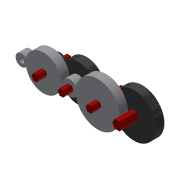
# Autodesk Inventor part: MultiStage Gearbox Sketch Double File
Saved by Autodesk Inventor 2013 (Build 170138000, 138)
## iProperties
Created: 2014-01-26
Part Number: MultiStage Gearbox Sketch Double File
Material: Generic
Document SubType Name: Modeling
Designer: Nemo
Density: 1 g/cm^3
Author: Nemo
Autodesk Inventor part; units mm, degrees
ref_plane "YZ Plane" through (0, 0, 0) normal (1, 0, 0) x (0, 1, 0)
ref_plane "XZ Plane" through (0, 0, 0) normal (0, 1, 0) x (-1, 0, 0)
ref_plane "XY Plane" through (0, 0, 0) normal (0, 0, 1) x (1, 0, 0)
sketch "Sketch1" plane through (0, 0, 0) normal (0, 0, 1) x (1, 0, 0)
  circle A0 centre (0, 0) radius 26.67
  line L0 (5.4993, 0) -> (2.7496, -4.7625)
  line L1 (2.7496, -4.7625) -> (-2.7496, -4.7625)
  line L2 (-2.7496, -4.7625) -> (-5.4993, 0)
  line L3 (-5.4993, 0) -> (-2.7496, 4.7625)
  line L4 (-2.7496, 4.7625) -> (2.7496, 4.7625)
  line L5 (2.7496, 4.7625) -> (5.4993, 0)
  circle A1 centre (0, 0) radius 13.97
  circle A2 centre (39.4462, 0) radius 27.94
  circle A3 centre (39.4462, 0) radius 11.43
  circle A4 centre (-33.0962, 0) radius 8.89
  circle A5 centre (81.4324, 0) radius 33.02
  line L6 (78.6828, 4.7625) -> (84.182, 4.7625)
  line L7 (84.182, 4.7625) -> (86.9317, 0)
  line L8 (86.9317, 0) -> (84.182, -4.7625)
  line L9 (84.182, -4.7625) -> (78.6828, -4.7625)
  line L10 (78.6828, -4.7625) -> (75.9331, 0)
  line L11 (75.9331, 0) -> (78.6828, 4.7625)
  line L12 (33.9469, 0) -> (36.6966, 4.7625)
  line L13 (36.6966, 4.7625) -> (42.1958, 4.7625)
  line L14 (42.1958, 4.7625) -> (44.9455, 0)
  line L15 (44.9455, 0) -> (42.1958, -4.7625)
  line L16 (42.1958, -4.7625) -> (36.6966, -4.7625)
  line L17 (36.6966, -4.7625) -> (33.9469, 0)
  circle A6 centre (-33.0962, 0) radius 4
  line L18 (-34.0962, 4.873) -> (-32.0962, 4.873)
  line L19 (-32.0962, 4.873) -> (-32.0962, 2.873)
  line L20 (-32.0962, 2.873) -> (-34.0962, 2.873)
  line L21 (-34.0962, 2.873) -> (-34.0962, 4.873)
  circle A7 centre (81.4324, 0) radius 11.43
  circle A8 centre (123.4186, 0) radius 33.02
  line L22 (127.0848, 6.35) -> (130.7509, 0)
  line L23 (130.7509, 0) -> (127.0848, -6.35)
  line L24 (127.0848, -6.35) -> (119.7524, -6.35)
  line L25 (119.7524, -6.35) -> (116.0863, 0)
  line L26 (116.0863, 0) -> (119.7524, 6.35)
  line L27 (119.7524, 6.35) -> (127.0848, 6.35)
  point P0 (-34.0962, 3.873)
  point P1 (-33.0962, 4.873)
  dimension "d18" = 8
  dimension "d0" = 53.34
  dimension "d1" = 9.525
  dimension "d2" = 27.94
  dimension "d3" = 55.88
  dimension "d4" = 39.4462
  dimension "d5" = 22.86
  dimension "d6" = 17.78
  dimension "d7" = 33.0962
  dimension "d8" = 66.04
  dimension "d9" = 41.9862
  dimension "d10" = 9.525
  dimension "d15" = 9.525
  dimension "d19" = 2
  dimension "d20" = 2
  dimension "d21" = 22.86
  dimension "d22" = 66.04
  dimension "d23" = 41.9862
  dimension "d24" = 12.7
  constraints: 56 end point, 9 coincident, 8 centre point, 6 horizontal alignment, 3 horizontal, 2 midpoint, 2 parallel, 1 perpendicular, 1 vertical alignment, 55 other
  measures "d0" diameter of A0
  measures "d1" distance between parallel lines of L1 L4
  measures "d2" diameter of A1
  measures "d3" diameter of A2
  measures "d4" distance of point (0, 0) A2.centre
  measures "d5" diameter of A3
  measures "d6" diameter of A4
  measures "d7" distance of point (0, 0) A4.centre
  measures "d8" diameter of A5
  measures "d9" distance of A5.centre A2.centre
  measures "d10" distance between parallel lines of L9 L6
  measures "d15" distance between parallel lines of L16 L13
  measures "d19" distance of L19.end L20.end
  measures "d20" distance of L18.end L19.end
  measures "d21" diameter of A7
  measures "d22" diameter of A8
  measures "d23" distance of A8.centre A5.centre
  measures "d24" distance between parallel lines of L24 L27
extrude "Extrusion1" add sketch "Sketch1" along normal blind 12.7 contours A0 A2 A1 | A2 A1 A0 A4 | A4 A0 | A0 A4 | A5 A8 A7 A2 | A2 A5 A3 | A2 A1 | A1 A2 | A5 A8 A7 | A5 A3 | A3 A5 | A8 A7 | A7 A8 | L0 L1 L2 L3 L4 L5
extrude "Extrusion2" add sketch "Sketch1" against normal blind 12.7 separate body contours A0 A2 A1 | A0 A2 A5 A3 | A2 A5 A3 | A2 A1 | A1 A2 | A8 A5 | A5 A8 A7 | A5 A3 | A3 A5 | A8 A7 | A7 A8 | L12 L13 L14 L15 L16 L17
extrude "Extrusion3" add sketch "Sketch1" along normal mid plane 50.8 separate body contours L0 L1 L2 L3 L4 L5 | L6 L7 L8 L9 L10 L11 | L12 L13 L14 L15 L16 L17 | L22 L23 L24 L25 L26 L27
equation "\"in1\" = 304.8"
equation "\"out1\" = 1016"
equation "\"in2\" = 508"
equation "\"out2\" = 1066.8"
equation "\"in3\" = 406.4"
equation "\"in4\" = 406.4"
body "Solid1"
body "Solid2"
body "Solid3"
